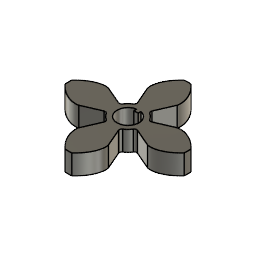
Gear 3 (Autodesk Fusion 360 design; units mm, degrees)
description: Spur Gear; Module: 12.700000; Num Teeth: 4; Pressure Angle: 20.000000; Backlash: 0.00 mm
Autodesk Fusion 360 part; units mm, degrees
sketch "Sketch1" plane through (0, 0, 0) normal (0, 0, 1) x (1, 0, 0) in component "Spur Gear (4 teeth)"
  circle A0 centre (0, 0) radius 10.1092
  circle A1 centre (0, 0) radius 6.35
extrude "Extrude1" add sketch "Sketch1" along normal blind 12.7 in component "Spur Gear (4 teeth)"
sketch "Sketch2" plane through (0, 0, 0) normal (0, 0, 1) x (1, 0, 0) in component "Spur Gear (4 teeth)"
  spline S0 degree 5 poles (21.9128, -9.4616) (21.9552, -9.4799) (22.0407, -9.5141) (22.1712, -9.5583) (22.3491, -9.6037) (22.5768, -9.6426) (22.8081, -9.6692) (23.0414, -9.6889) (23.2758, -9.7048) (23.5109, -9.7174) (23.7467, -9.7262) (23.9837, -9.7295) (24.2219, -9.7262) (24.4615, -9.7158) (24.7023, -9.6987) (24.9439, -9.6758) (25.1862, -9.648) (25.4288, -9.6159) (25.6717, -9.5798) (25.9149, -9.5397) (26.1582, -9.4952) (26.4018, -9.4462) (26.6456, -9.3926) (26.8896, -9.3344) (27.1337, -9.2719) (27.3777, -9.2051) (27.6217, -9.1343) (27.8655, -9.0596) (28.109, -8.9811) (28.3523, -8.8987) (28.5954, -8.8125) (28.838, -8.7225) (29.0803, -8.6286) (29.3222, -8.531) (29.5637, -8.4296) (29.8046, -8.3246) (30.045, -8.216) (30.2848, -8.1038) (30.5239, -7.9882) (30.7623, -7.869) (31.0001, -7.7465) (31.2371, -7.6205) (31.4733, -7.491) (31.7087, -7.3583) (31.9432, -7.2221) (32.1769, -7.0827) (32.4096, -6.9401) (32.6414, -6.7942) (32.8722, -6.6451) (33.1019, -6.4928) (33.3306, -6.3374) (33.5583, -6.1789) (33.7848, -6.0173) (34.0102, -5.8526) (34.2343, -5.6849) (34.4573, -5.5142) (34.6791, -5.3405) (34.8996, -5.1639) (35.1188, -4.9843) (35.3367, -4.8018) (35.5532, -4.6165) (35.7684, -4.4283) (35.9823, -4.2373) (36.1947, -4.0436) (36.4056, -3.847) (36.6151, -3.6477) (36.823, -3.4457) (37.0294, -3.241) (37.2343, -3.0337) (37.4376, -2.8237) (37.6393, -2.6111) (37.7995, -2.4389) (37.9189, -2.3086) (37.9982, -2.2212) (38.0377, -2.1774) knots 0 0 0 0 0 0 0.01428571 0.02857143 0.04285714 0.05714286 0.07142857 0.08571429 0.1 0.11428571 0.12857143 0.14285714 0.15714286 0.17142857 0.18571429 0.2 0.21428571 0.22857143 0.24285714 0.25714286 0.27142857 0.28571429 0.3 0.31428571 0.32857143 0.34285714 0.35714286 0.37142857 0.38571429 0.4 0.41428571 0.42857143 0.44285714 0.45714286 0.47142857 0.48571429 0.5 0.51428571 0.52857143 0.54285714 0.55714286 0.57142857 0.58571429 0.6 0.61428571 0.62857143 0.64285714 0.65714286 0.67142857 0.68571429 0.7 0.71428571 0.72857143 0.74285714 0.75714286 0.77142857 0.78571429 0.8 0.81428571 0.82857143 0.84285714 0.85714286 0.87142857 0.88571429 0.9 0.91428571 0.92857143 0.94285714 0.95714286 0.97142857 0.98571429 1 1 1 1 1 1
  spline S1 degree 5 poles (21.9128, 9.4616) (21.9552, 9.4799) (22.0407, 9.5141) (22.1712, 9.5583) (22.3491, 9.6037) (22.5768, 9.6426) (22.8081, 9.6692) (23.0414, 9.6889) (23.2758, 9.7048) (23.5109, 9.7174) (23.7467, 9.7262) (23.9837, 9.7295) (24.2219, 9.7262) (24.4615, 9.7158) (24.7023, 9.6987) (24.9439, 9.6758) (25.1862, 9.648) (25.4288, 9.6159) (25.6717, 9.5798) (25.9149, 9.5397) (26.1582, 9.4952) (26.4018, 9.4462) (26.6456, 9.3926) (26.8896, 9.3344) (27.1337, 9.2719) (27.3777, 9.2051) (27.6217, 9.1343) (27.8655, 9.0596) (28.109, 8.9811) (28.3523, 8.8987) (28.5954, 8.8125) (28.838, 8.7225) (29.0803, 8.6286) (29.3222, 8.531) (29.5637, 8.4296) (29.8046, 8.3246) (30.045, 8.216) (30.2848, 8.1038) (30.5239, 7.9882) (30.7623, 7.869) (31.0001, 7.7465) (31.2371, 7.6205) (31.4733, 7.491) (31.7087, 7.3583) (31.9432, 7.2221) (32.1769, 7.0827) (32.4096, 6.9401) (32.6414, 6.7942) (32.8722, 6.6451) (33.1019, 6.4928) (33.3306, 6.3374) (33.5583, 6.1789) (33.7848, 6.0173) (34.0102, 5.8526) (34.2343, 5.6849) (34.4573, 5.5142) (34.6791, 5.3405) (34.8996, 5.1639) (35.1188, 4.9843) (35.3367, 4.8018) (35.5532, 4.6165) (35.7684, 4.4283) (35.9823, 4.2373) (36.1947, 4.0436) (36.4056, 3.847) (36.6151, 3.6477) (36.823, 3.4457) (37.0294, 3.241) (37.2343, 3.0337) (37.4376, 2.8237) (37.6393, 2.6111) (37.7995, 2.4389) (37.9189, 2.3086) (37.9982, 2.2212) (38.0377, 2.1774) knots 0 0 0 0 0 0 0.01428571 0.02857143 0.04285714 0.05714286 0.07142857 0.08571429 0.1 0.11428571 0.12857143 0.14285714 0.15714286 0.17142857 0.18571429 0.2 0.21428571 0.22857143 0.24285714 0.25714286 0.27142857 0.28571429 0.3 0.31428571 0.32857143 0.34285714 0.35714286 0.37142857 0.38571429 0.4 0.41428571 0.42857143 0.44285714 0.45714286 0.47142857 0.48571429 0.5 0.51428571 0.52857143 0.54285714 0.55714286 0.57142857 0.58571429 0.6 0.61428571 0.62857143 0.64285714 0.65714286 0.67142857 0.68571429 0.7 0.71428571 0.72857143 0.74285714 0.75714286 0.77142857 0.78571429 0.8 0.81428571 0.82857143 0.84285714 0.85714286 0.87142857 0.88571429 0.9 0.91428571 0.92857143 0.94285714 0.95714286 0.97142857 0.98571429 1 1 1 1 1 1
  arc A0 (38.0377, -2.1774) -> (38.0377, 2.1774) centre (0, 0) ccw
  line L0 (9.2718, -4.0074) -> (21.9128, -9.4616)
  line L1 (9.2718, 4.0074) -> (21.9128, 9.4616)
  line L2 (9.2718, -4.0074) -> (9.2718, 4.0074)
  point P0 (22.9255, -9.6784)
  point P1 (24.0052, -9.7278)
  point P2 (25.1271, -9.6541)
  point P3 (26.2802, -9.4701)
  point P4 (27.4564, -9.1817)
  point P5 (28.6488, -8.792)
  point P6 (29.8509, -8.303)
  point P7 (31.0565, -7.7159)
  point P8 (32.2598, -7.0314)
  point P9 (33.4549, -6.2504)
  point P10 (34.636, -5.3736)
  point P11 (35.7973, -4.4018)
  point P12 (36.9331, -3.336)
  point P13 (22.9255, 9.6784)
  point P14 (24.0052, 9.7278)
  point P15 (25.1271, 9.6541)
  point P16 (26.2802, 9.4701)
  point P17 (27.4564, 9.1817)
  point P18 (28.6488, 8.792)
  point P19 (29.8509, 8.303)
  point P20 (31.0565, 7.7159)
  point P21 (32.2598, 7.0314)
  point P22 (33.4549, 6.2504)
  point P23 (34.636, 5.3736)
  point P24 (35.7973, 4.4018)
  point P25 (36.9331, 3.336)
extrude "Extrude2" add sketch "Sketch2" along normal blind 12.7 in component "Spur Gear (4 teeth)"
fillet "Fillet1" radius 1.5875 2 edges at (9.2795, -4.0107, 6.35) (9.2795, 4.0107, 6.35) in component "Spur Gear (4 teeth)"
pattern_circular "C-Pattern1" count 4 over 360 about axis through (0, 0, 0) along (0, 0, 1) of "Extrude2", "Fillet1" in component "Spur Gear (4 teeth)"
sketch "Sketch3" plane through (0, 0, 0) normal (0, 0, 1) x (1, 0, 0) in component "Spur Gear (4 teeth)"
  circle A0 centre (0, 0) radius 25.4 construction
sketch "Sketch1 (2)" plane through (0, 0, 12.7) normal (0, 0, 1) x (-1, 0, 0)
  arc A0 (-5.2324, 8.6498) -> (-8.6498, 5.2324) centre (0, 0) ccw
  arc A1 (-10.637, 4.5964) -> (-8.6498, 5.2324) centre (-10.0081, 6.054) ccw
  line L0 (-10.637, 4.5964) -> (-21.9128, 9.4616)
  spline S0 degree 5 poles (-21.9128, 9.4616) (-21.9552, 9.4799) (-22.0407, 9.5141) (-22.1712, 9.5583) (-22.3491, 9.6037) (-22.5768, 9.6426) (-22.8081, 9.6692) (-23.0414, 9.6889) (-23.2758, 9.7048) (-23.5109, 9.7174) (-23.7467, 9.7262) (-23.9837, 9.7295) (-24.2219, 9.7262) (-24.4615, 9.7158) (-24.7023, 9.6987) (-24.9439, 9.6758) (-25.1862, 9.648) (-25.4288, 9.6159) (-25.6717, 9.5798) (-25.9149, 9.5397) (-26.1582, 9.4952) (-26.4018, 9.4462) (-26.6456, 9.3926) (-26.8896, 9.3344) (-27.1337, 9.2719) (-27.3777, 9.2051) (-27.6217, 9.1343) (-27.8655, 9.0596) (-28.109, 8.9811) (-28.3523, 8.8987) (-28.5954, 8.8125) (-28.838, 8.7225) (-29.0803, 8.6286) (-29.3222, 8.531) (-29.5637, 8.4296) (-29.8046, 8.3246) (-30.045, 8.216) (-30.2848, 8.1038) (-30.5239, 7.9882) (-30.7623, 7.869) (-31.0001, 7.7465) (-31.2371, 7.6205) (-31.4733, 7.491) (-31.7087, 7.3583) (-31.9432, 7.2221) (-32.1769, 7.0827) (-32.4096, 6.9401) (-32.6414, 6.7942) (-32.8722, 6.6451) (-33.1019, 6.4928) (-33.3306, 6.3374) (-33.5583, 6.1789) (-33.7848, 6.0173) (-34.0102, 5.8526) (-34.2343, 5.6849) (-34.4573, 5.5142) (-34.6791, 5.3405) (-34.8996, 5.1639) (-35.1188, 4.9843) (-35.3367, 4.8018) (-35.5532, 4.6165) (-35.7684, 4.4283) (-35.9823, 4.2373) (-36.1947, 4.0436) (-36.4056, 3.847) (-36.6151, 3.6477) (-36.823, 3.4457) (-37.0294, 3.241) (-37.2343, 3.0337) (-37.4376, 2.8237) (-37.6393, 2.6111) (-37.7995, 2.4389) (-37.9189, 2.3086) (-37.9982, 2.2212) (-38.0377, 2.1774) knots 0 0 0 0 0 0 0.01428571 0.02857143 0.04285714 0.05714286 0.07142857 0.08571429 0.1 0.11428571 0.12857143 0.14285714 0.15714286 0.17142857 0.18571429 0.2 0.21428571 0.22857143 0.24285714 0.25714286 0.27142857 0.28571429 0.3 0.31428571 0.32857143 0.34285714 0.35714286 0.37142857 0.38571429 0.4 0.41428571 0.42857143 0.44285714 0.45714286 0.47142857 0.48571429 0.5 0.51428571 0.52857143 0.54285714 0.55714286 0.57142857 0.58571429 0.6 0.61428571 0.62857143 0.64285714 0.65714286 0.67142857 0.68571429 0.7 0.71428571 0.72857143 0.74285714 0.75714286 0.77142857 0.78571429 0.8 0.81428571 0.82857143 0.84285714 0.85714286 0.87142857 0.88571429 0.9 0.91428571 0.92857143 0.94285714 0.95714286 0.97142857 0.98571429 1 1 1 1 1 1
  arc A2 (-38.0377, 2.1774) -> (-38.0377, -2.1774) centre (0, 0) ccw
  spline S1 degree 5 poles (-38.0377, -2.1774) (-37.9982, -2.2212) (-37.9189, -2.3086) (-37.7995, -2.4389) (-37.6393, -2.6111) (-37.4376, -2.8237) (-37.2343, -3.0337) (-37.0294, -3.241) (-36.823, -3.4457) (-36.6151, -3.6477) (-36.4056, -3.847) (-36.1947, -4.0436) (-35.9823, -4.2373) (-35.7684, -4.4283) (-35.5532, -4.6165) (-35.3367, -4.8018) (-35.1188, -4.9843) (-34.8996, -5.1639) (-34.6791, -5.3405) (-34.4573, -5.5142) (-34.2343, -5.6849) (-34.0102, -5.8526) (-33.7848, -6.0173) (-33.5583, -6.1789) (-33.3306, -6.3374) (-33.1019, -6.4928) (-32.8722, -6.6451) (-32.6414, -6.7942) (-32.4096, -6.9401) (-32.1769, -7.0827) (-31.9432, -7.2221) (-31.7087, -7.3583) (-31.4733, -7.491) (-31.2371, -7.6205) (-31.0001, -7.7465) (-30.7623, -7.869) (-30.5239, -7.9882) (-30.2848, -8.1038) (-30.045, -8.216) (-29.8046, -8.3246) (-29.5637, -8.4296) (-29.3222, -8.531) (-29.0803, -8.6286) (-28.838, -8.7225) (-28.5954, -8.8125) (-28.3523, -8.8987) (-28.109, -8.9811) (-27.8655, -9.0596) (-27.6217, -9.1343) (-27.3777, -9.2051) (-27.1337, -9.2719) (-26.8896, -9.3344) (-26.6456, -9.3926) (-26.4018, -9.4462) (-26.1582, -9.4952) (-25.9149, -9.5397) (-25.6717, -9.5798) (-25.4288, -9.6159) (-25.1862, -9.648) (-24.9439, -9.6758) (-24.7023, -9.6987) (-24.4615, -9.7158) (-24.2219, -9.7262) (-23.9837, -9.7295) (-23.7467, -9.7262) (-23.5109, -9.7174) (-23.2758, -9.7048) (-23.0414, -9.6889) (-22.8081, -9.6692) (-22.5768, -9.6426) (-22.3491, -9.6037) (-22.1712, -9.5583) (-22.0407, -9.5141) (-21.9552, -9.4799) (-21.9128, -9.4616) knots -1 -1 -1 -1 -1 -1 -0.98571429 -0.97142857 -0.95714286 -0.94285714 -0.92857143 -0.91428571 -0.9 -0.88571429 -0.87142857 -0.85714286 -0.84285714 -0.82857143 -0.81428571 -0.8 -0.78571429 -0.77142857 -0.75714286 -0.74285714 -0.72857143 -0.71428571 -0.7 -0.68571429 -0.67142857 -0.65714286 -0.64285714 -0.62857143 -0.61428571 -0.6 -0.58571429 -0.57142857 -0.55714286 -0.54285714 -0.52857143 -0.51428571 -0.5 -0.48571429 -0.47142857 -0.45714286 -0.44285714 -0.42857143 -0.41428571 -0.4 -0.38571429 -0.37142857 -0.35714286 -0.34285714 -0.32857143 -0.31428571 -0.3 -0.28571429 -0.27142857 -0.25714286 -0.24285714 -0.22857143 -0.21428571 -0.2 -0.18571429 -0.17142857 -0.15714286 -0.14285714 -0.12857143 -0.11428571 -0.1 -0.08571429 -0.07142857 -0.05714286 -0.04285714 -0.02857143 -0.01428571 0 0 0 0 0 0
  line L1 (-21.9128, -9.4616) -> (-10.637, -4.5964)
  arc A3 (-8.6498, -5.2324) -> (-10.637, -4.5964) centre (-10.0081, -6.054) ccw
  arc A4 (-8.6498, -5.2324) -> (-5.2324, -8.6498) centre (0, 0) ccw
  arc A5 (-4.5964, -10.637) -> (-5.2324, -8.6498) centre (-6.054, -10.0081) ccw
  line L2 (-4.5964, -10.637) -> (-9.4616, -21.9128)
  spline S2 degree 5 poles (-9.4616, -21.9128) (-9.4799, -21.9552) (-9.5141, -22.0407) (-9.5583, -22.1712) (-9.6037, -22.3491) (-9.6426, -22.5768) (-9.6692, -22.8081) (-9.6889, -23.0414) (-9.7048, -23.2758) (-9.7174, -23.5109) (-9.7262, -23.7467) (-9.7295, -23.9837) (-9.7262, -24.2219) (-9.7158, -24.4615) (-9.6987, -24.7023) (-9.6758, -24.9439) (-9.648, -25.1862) (-9.6159, -25.4288) (-9.5798, -25.6717) (-9.5397, -25.9149) (-9.4952, -26.1582) (-9.4462, -26.4018) (-9.3926, -26.6456) (-9.3344, -26.8896) (-9.2719, -27.1337) (-9.2051, -27.3777) (-9.1343, -27.6217) (-9.0596, -27.8655) (-8.9811, -28.109) (-8.8987, -28.3523) (-8.8125, -28.5954) (-8.7225, -28.838) (-8.6286, -29.0803) (-8.531, -29.3222) (-8.4296, -29.5637) (-8.3246, -29.8046) (-8.216, -30.045) (-8.1038, -30.2848) (-7.9882, -30.5239) (-7.869, -30.7623) (-7.7465, -31.0001) (-7.6205, -31.2371) (-7.491, -31.4733) (-7.3583, -31.7087) (-7.2221, -31.9432) (-7.0827, -32.1769) (-6.9401, -32.4096) (-6.7942, -32.6414) (-6.6451, -32.8722) (-6.4928, -33.1019) (-6.3374, -33.3306) (-6.1789, -33.5583) (-6.0173, -33.7848) (-5.8526, -34.0102) (-5.6849, -34.2343) (-5.5142, -34.4573) (-5.3405, -34.6791) (-5.1639, -34.8996) (-4.9843, -35.1188) (-4.8018, -35.3367) (-4.6165, -35.5532) (-4.4283, -35.7684) (-4.2373, -35.9823) (-4.0436, -36.1947) (-3.847, -36.4056) (-3.6477, -36.6151) (-3.4457, -36.823) (-3.241, -37.0294) (-3.0337, -37.2343) (-2.8237, -37.4376) (-2.6111, -37.6393) (-2.4389, -37.7995) (-2.3086, -37.9189) (-2.2212, -37.9982) (-2.1774, -38.0377) knots 0 0 0 0 0 0 0.01428571 0.02857143 0.04285714 0.05714286 0.07142857 0.08571429 0.1 0.11428571 0.12857143 0.14285714 0.15714286 0.17142857 0.18571429 0.2 0.21428571 0.22857143 0.24285714 0.25714286 0.27142857 0.28571429 0.3 0.31428571 0.32857143 0.34285714 0.35714286 0.37142857 0.38571429 0.4 0.41428571 0.42857143 0.44285714 0.45714286 0.47142857 0.48571429 0.5 0.51428571 0.52857143 0.54285714 0.55714286 0.57142857 0.58571429 0.6 0.61428571 0.62857143 0.64285714 0.65714286 0.67142857 0.68571429 0.7 0.71428571 0.72857143 0.74285714 0.75714286 0.77142857 0.78571429 0.8 0.81428571 0.82857143 0.84285714 0.85714286 0.87142857 0.88571429 0.9 0.91428571 0.92857143 0.94285714 0.95714286 0.97142857 0.98571429 1 1 1 1 1 1
  arc A6 (-2.1774, -38.0377) -> (2.1774, -38.0377) centre (0, 0) ccw
  spline S3 degree 5 poles (2.1774, -38.0377) (2.2212, -37.9982) (2.3086, -37.9189) (2.4389, -37.7995) (2.6111, -37.6393) (2.8237, -37.4376) (3.0337, -37.2343) (3.241, -37.0294) (3.4457, -36.823) (3.6477, -36.6151) (3.847, -36.4056) (4.0436, -36.1947) (4.2373, -35.9823) (4.4283, -35.7684) (4.6165, -35.5532) (4.8018, -35.3367) (4.9843, -35.1188) (5.1639, -34.8996) (5.3405, -34.6791) (5.5142, -34.4573) (5.6849, -34.2343) (5.8526, -34.0102) (6.0173, -33.7848) (6.1789, -33.5583) (6.3374, -33.3306) (6.4928, -33.1019) (6.6451, -32.8722) (6.7942, -32.6414) (6.9401, -32.4096) (7.0827, -32.1769) (7.2221, -31.9432) (7.3583, -31.7087) (7.491, -31.4733) (7.6205, -31.2371) (7.7465, -31.0001) (7.869, -30.7623) (7.9882, -30.5239) (8.1038, -30.2848) (8.216, -30.045) (8.3246, -29.8046) (8.4296, -29.5637) (8.531, -29.3222) (8.6286, -29.0803) (8.7225, -28.838) (8.8125, -28.5954) (8.8987, -28.3523) (8.9811, -28.109) (9.0596, -27.8655) (9.1343, -27.6217) (9.2051, -27.3777) (9.2719, -27.1337) (9.3344, -26.8896) (9.3926, -26.6456) (9.4462, -26.4018) (9.4952, -26.1582) (9.5397, -25.9149) (9.5798, -25.6717) (9.6159, -25.4288) (9.648, -25.1862) (9.6758, -24.9439) (9.6987, -24.7023) (9.7158, -24.4615) (9.7262, -24.2219) (9.7295, -23.9837) (9.7262, -23.7467) (9.7174, -23.5109) (9.7048, -23.2758) (9.6889, -23.0414) (9.6692, -22.8081) (9.6426, -22.5768) (9.6037, -22.3491) (9.5583, -22.1712) (9.5141, -22.0407) (9.4799, -21.9552) (9.4616, -21.9128) knots -1 -1 -1 -1 -1 -1 -0.98571429 -0.97142857 -0.95714286 -0.94285714 -0.92857143 -0.91428571 -0.9 -0.88571429 -0.87142857 -0.85714286 -0.84285714 -0.82857143 -0.81428571 -0.8 -0.78571429 -0.77142857 -0.75714286 -0.74285714 -0.72857143 -0.71428571 -0.7 -0.68571429 -0.67142857 -0.65714286 -0.64285714 -0.62857143 -0.61428571 -0.6 -0.58571429 -0.57142857 -0.55714286 -0.54285714 -0.52857143 -0.51428571 -0.5 -0.48571429 -0.47142857 -0.45714286 -0.44285714 -0.42857143 -0.41428571 -0.4 -0.38571429 -0.37142857 -0.35714286 -0.34285714 -0.32857143 -0.31428571 -0.3 -0.28571429 -0.27142857 -0.25714286 -0.24285714 -0.22857143 -0.21428571 -0.2 -0.18571429 -0.17142857 -0.15714286 -0.14285714 -0.12857143 -0.11428571 -0.1 -0.08571429 -0.07142857 -0.05714286 -0.04285714 -0.02857143 -0.01428571 0 0 0 0 0 0
  line L3 (9.4616, -21.9128) -> (4.5964, -10.637)
  arc A7 (5.2324, -8.6498) -> (4.5964, -10.637) centre (6.054, -10.0081) ccw
  arc A8 (5.2324, -8.6498) -> (8.6498, -5.2324) centre (0, 0) ccw
  arc A9 (10.637, -4.5964) -> (8.6498, -5.2324) centre (10.0081, -6.054) ccw
  line L4 (10.637, -4.5964) -> (21.9128, -9.4616)
  spline S4 degree 5 poles (21.9128, -9.4616) (21.9552, -9.4799) (22.0407, -9.5141) (22.1712, -9.5583) (22.3491, -9.6037) (22.5768, -9.6426) (22.8081, -9.6692) (23.0414, -9.6889) (23.2758, -9.7048) (23.5109, -9.7174) (23.7467, -9.7262) (23.9837, -9.7295) (24.2219, -9.7262) (24.4615, -9.7158) (24.7023, -9.6987) (24.9439, -9.6758) (25.1862, -9.648) (25.4288, -9.6159) (25.6717, -9.5798) (25.9149, -9.5397) (26.1582, -9.4952) (26.4018, -9.4462) (26.6456, -9.3926) (26.8896, -9.3344) (27.1337, -9.2719) (27.3777, -9.2051) (27.6217, -9.1343) (27.8655, -9.0596) (28.109, -8.9811) (28.3523, -8.8987) (28.5954, -8.8125) (28.838, -8.7225) (29.0803, -8.6286) (29.3222, -8.531) (29.5637, -8.4296) (29.8046, -8.3246) (30.045, -8.216) (30.2848, -8.1038) (30.5239, -7.9882) (30.7623, -7.869) (31.0001, -7.7465) (31.2371, -7.6205) (31.4733, -7.491) (31.7087, -7.3583) (31.9432, -7.2221) (32.1769, -7.0827) (32.4096, -6.9401) (32.6414, -6.7942) (32.8722, -6.6451) (33.1019, -6.4928) (33.3306, -6.3374) (33.5583, -6.1789) (33.7848, -6.0173) (34.0102, -5.8526) (34.2343, -5.6849) (34.4573, -5.5142) (34.6791, -5.3405) (34.8996, -5.1639) (35.1188, -4.9843) (35.3367, -4.8018) (35.5532, -4.6165) (35.7684, -4.4283) (35.9823, -4.2373) (36.1947, -4.0436) (36.4056, -3.847) (36.6151, -3.6477) (36.823, -3.4457) (37.0294, -3.241) (37.2343, -3.0337) (37.4376, -2.8237) (37.6393, -2.6111) (37.7995, -2.4389) (37.9189, -2.3086) (37.9982, -2.2212) (38.0377, -2.1774) knots 0 0 0 0 0 0 0.01428571 0.02857143 0.04285714 0.05714286 0.07142857 0.08571429 0.1 0.11428571 0.12857143 0.14285714 0.15714286 0.17142857 0.18571429 0.2 0.21428571 0.22857143 0.24285714 0.25714286 0.27142857 0.28571429 0.3 0.31428571 0.32857143 0.34285714 0.35714286 0.37142857 0.38571429 0.4 0.41428571 0.42857143 0.44285714 0.45714286 0.47142857 0.48571429 0.5 0.51428571 0.52857143 0.54285714 0.55714286 0.57142857 0.58571429 0.6 0.61428571 0.62857143 0.64285714 0.65714286 0.67142857 0.68571429 0.7 0.71428571 0.72857143 0.74285714 0.75714286 0.77142857 0.78571429 0.8 0.81428571 0.82857143 0.84285714 0.85714286 0.87142857 0.88571429 0.9 0.91428571 0.92857143 0.94285714 0.95714286 0.97142857 0.98571429 1 1 1 1 1 1
  arc A10 (38.0377, -2.1774) -> (38.0377, 2.1774) centre (0, 0) ccw
  spline S5 degree 5 poles (38.0377, 2.1774) (37.9982, 2.2212) (37.9189, 2.3086) (37.7995, 2.4389) (37.6393, 2.6111) (37.4376, 2.8237) (37.2343, 3.0337) (37.0294, 3.241) (36.823, 3.4457) (36.6151, 3.6477) (36.4056, 3.847) (36.1947, 4.0436) (35.9823, 4.2373) (35.7684, 4.4283) (35.5532, 4.6165) (35.3367, 4.8018) (35.1188, 4.9843) (34.8996, 5.1639) (34.6791, 5.3405) (34.4573, 5.5142) (34.2343, 5.6849) (34.0102, 5.8526) (33.7848, 6.0173) (33.5583, 6.1789) (33.3306, 6.3374) (33.1019, 6.4928) (32.8722, 6.6451) (32.6414, 6.7942) (32.4096, 6.9401) (32.1769, 7.0827) (31.9432, 7.2221) (31.7087, 7.3583) (31.4733, 7.491) (31.2371, 7.6205) (31.0001, 7.7465) (30.7623, 7.869) (30.5239, 7.9882) (30.2848, 8.1038) (30.045, 8.216) (29.8046, 8.3246) (29.5637, 8.4296) (29.3222, 8.531) (29.0803, 8.6286) (28.838, 8.7225) (28.5954, 8.8125) (28.3523, 8.8987) (28.109, 8.9811) (27.8655, 9.0596) (27.6217, 9.1343) (27.3777, 9.2051) (27.1337, 9.2719) (26.8896, 9.3344) (26.6456, 9.3926) (26.4018, 9.4462) (26.1582, 9.4952) (25.9149, 9.5397) (25.6717, 9.5798) (25.4288, 9.6159) (25.1862, 9.648) (24.9439, 9.6758) (24.7023, 9.6987) (24.4615, 9.7158) (24.2219, 9.7262) (23.9837, 9.7295) (23.7467, 9.7262) (23.5109, 9.7174) (23.2758, 9.7048) (23.0414, 9.6889) (22.8081, 9.6692) (22.5768, 9.6426) (22.3491, 9.6037) (22.1712, 9.5583) (22.0407, 9.5141) (21.9552, 9.4799) (21.9128, 9.4616) knots -1 -1 -1 -1 -1 -1 -0.98571429 -0.97142857 -0.95714286 -0.94285714 -0.92857143 -0.91428571 -0.9 -0.88571429 -0.87142857 -0.85714286 -0.84285714 -0.82857143 -0.81428571 -0.8 -0.78571429 -0.77142857 -0.75714286 -0.74285714 -0.72857143 -0.71428571 -0.7 -0.68571429 -0.67142857 -0.65714286 -0.64285714 -0.62857143 -0.61428571 -0.6 -0.58571429 -0.57142857 -0.55714286 -0.54285714 -0.52857143 -0.51428571 -0.5 -0.48571429 -0.47142857 -0.45714286 -0.44285714 -0.42857143 -0.41428571 -0.4 -0.38571429 -0.37142857 -0.35714286 -0.34285714 -0.32857143 -0.31428571 -0.3 -0.28571429 -0.27142857 -0.25714286 -0.24285714 -0.22857143 -0.21428571 -0.2 -0.18571429 -0.17142857 -0.15714286 -0.14285714 -0.12857143 -0.11428571 -0.1 -0.08571429 -0.07142857 -0.05714286 -0.04285714 -0.02857143 -0.01428571 0 0 0 0 0 0
  line L5 (21.9128, 9.4616) -> (10.637, 4.5964)
  arc A11 (8.6498, 5.2324) -> (10.637, 4.5964) centre (10.0081, 6.054) ccw
  arc A12 (8.6498, 5.2324) -> (5.2324, 8.6498) centre (0, 0) ccw
  arc A13 (4.5964, 10.637) -> (5.2324, 8.6498) centre (6.054, 10.0081) ccw
  line L6 (4.5964, 10.637) -> (9.4616, 21.9128)
  spline S6 degree 5 poles (9.4616, 21.9128) (9.4799, 21.9552) (9.5141, 22.0407) (9.5583, 22.1712) (9.6037, 22.3491) (9.6426, 22.5768) (9.6692, 22.8081) (9.6889, 23.0414) (9.7048, 23.2758) (9.7174, 23.5109) (9.7262, 23.7467) (9.7295, 23.9837) (9.7262, 24.2219) (9.7158, 24.4615) (9.6987, 24.7023) (9.6758, 24.9439) (9.648, 25.1862) (9.6159, 25.4288) (9.5798, 25.6717) (9.5397, 25.9149) (9.4952, 26.1582) (9.4462, 26.4018) (9.3926, 26.6456) (9.3344, 26.8896) (9.2719, 27.1337) (9.2051, 27.3777) (9.1343, 27.6217) (9.0596, 27.8655) (8.9811, 28.109) (8.8987, 28.3523) (8.8125, 28.5954) (8.7225, 28.838) (8.6286, 29.0803) (8.531, 29.3222) (8.4296, 29.5637) (8.3246, 29.8046) (8.216, 30.045) (8.1038, 30.2848) (7.9882, 30.5239) (7.869, 30.7623) (7.7465, 31.0001) (7.6205, 31.2371) (7.491, 31.4733) (7.3583, 31.7087) (7.2221, 31.9432) (7.0827, 32.1769) (6.9401, 32.4096) (6.7942, 32.6414) (6.6451, 32.8722) (6.4928, 33.1019) (6.3374, 33.3306) (6.1789, 33.5583) (6.0173, 33.7848) (5.8526, 34.0102) (5.6849, 34.2343) (5.5142, 34.4573) (5.3405, 34.6791) (5.1639, 34.8996) (4.9843, 35.1188) (4.8018, 35.3367) (4.6165, 35.5532) (4.4283, 35.7684) (4.2373, 35.9823) (4.0436, 36.1947) (3.847, 36.4056) (3.6477, 36.6151) (3.4457, 36.823) (3.241, 37.0294) (3.0337, 37.2343) (2.8237, 37.4376) (2.6111, 37.6393) (2.4389, 37.7995) (2.3086, 37.9189) (2.2212, 37.9982) (2.1774, 38.0377) knots 0 0 0 0 0 0 0.01428571 0.02857143 0.04285714 0.05714286 0.07142857 0.08571429 0.1 0.11428571 0.12857143 0.14285714 0.15714286 0.17142857 0.18571429 0.2 0.21428571 0.22857143 0.24285714 0.25714286 0.27142857 0.28571429 0.3 0.31428571 0.32857143 0.34285714 0.35714286 0.37142857 0.38571429 0.4 0.41428571 0.42857143 0.44285714 0.45714286 0.47142857 0.48571429 0.5 0.51428571 0.52857143 0.54285714 0.55714286 0.57142857 0.58571429 0.6 0.61428571 0.62857143 0.64285714 0.65714286 0.67142857 0.68571429 0.7 0.71428571 0.72857143 0.74285714 0.75714286 0.77142857 0.78571429 0.8 0.81428571 0.82857143 0.84285714 0.85714286 0.87142857 0.88571429 0.9 0.91428571 0.92857143 0.94285714 0.95714286 0.97142857 0.98571429 1 1 1 1 1 1
  arc A14 (2.1774, 38.0377) -> (-2.1774, 38.0377) centre (0, 0) ccw
  spline S7 degree 5 poles (-2.1774, 38.0377) (-2.2212, 37.9982) (-2.3086, 37.9189) (-2.4389, 37.7995) (-2.6111, 37.6393) (-2.8237, 37.4376) (-3.0337, 37.2343) (-3.241, 37.0294) (-3.4457, 36.823) (-3.6477, 36.6151) (-3.847, 36.4056) (-4.0436, 36.1947) (-4.2373, 35.9823) (-4.4283, 35.7684) (-4.6165, 35.5532) (-4.8018, 35.3367) (-4.9843, 35.1188) (-5.1639, 34.8996) (-5.3405, 34.6791) (-5.5142, 34.4573) (-5.6849, 34.2343) (-5.8526, 34.0102) (-6.0173, 33.7848) (-6.1789, 33.5583) (-6.3374, 33.3306) (-6.4928, 33.1019) (-6.6451, 32.8722) (-6.7942, 32.6414) (-6.9401, 32.4096) (-7.0827, 32.1769) (-7.2221, 31.9432) (-7.3583, 31.7087) (-7.491, 31.4733) (-7.6205, 31.2371) (-7.7465, 31.0001) (-7.869, 30.7623) (-7.9882, 30.5239) (-8.1038, 30.2848) (-8.216, 30.045) (-8.3246, 29.8046) (-8.4296, 29.5637) (-8.531, 29.3222) (-8.6286, 29.0803) (-8.7225, 28.838) (-8.8125, 28.5954) (-8.8987, 28.3523) (-8.9811, 28.109) (-9.0596, 27.8655) (-9.1343, 27.6217) (-9.2051, 27.3777) (-9.2719, 27.1337) (-9.3344, 26.8896) (-9.3926, 26.6456) (-9.4462, 26.4018) (-9.4952, 26.1582) (-9.5397, 25.9149) (-9.5798, 25.6717) (-9.6159, 25.4288) (-9.648, 25.1862) (-9.6758, 24.9439) (-9.6987, 24.7023) (-9.7158, 24.4615) (-9.7262, 24.2219) (-9.7295, 23.9837) (-9.7262, 23.7467) (-9.7174, 23.5109) (-9.7048, 23.2758) (-9.6889, 23.0414) (-9.6692, 22.8081) (-9.6426, 22.5768) (-9.6037, 22.3491) (-9.5583, 22.1712) (-9.5141, 22.0407) (-9.4799, 21.9552) (-9.4616, 21.9128) knots -1 -1 -1 -1 -1 -1 -0.98571429 -0.97142857 -0.95714286 -0.94285714 -0.92857143 -0.91428571 -0.9 -0.88571429 -0.87142857 -0.85714286 -0.84285714 -0.82857143 -0.81428571 -0.8 -0.78571429 -0.77142857 -0.75714286 -0.74285714 -0.72857143 -0.71428571 -0.7 -0.68571429 -0.67142857 -0.65714286 -0.64285714 -0.62857143 -0.61428571 -0.6 -0.58571429 -0.57142857 -0.55714286 -0.54285714 -0.52857143 -0.51428571 -0.5 -0.48571429 -0.47142857 -0.45714286 -0.44285714 -0.42857143 -0.41428571 -0.4 -0.38571429 -0.37142857 -0.35714286 -0.34285714 -0.32857143 -0.31428571 -0.3 -0.28571429 -0.27142857 -0.25714286 -0.24285714 -0.22857143 -0.21428571 -0.2 -0.18571429 -0.17142857 -0.15714286 -0.14285714 -0.12857143 -0.11428571 -0.1 -0.08571429 -0.07142857 -0.05714286 -0.04285714 -0.02857143 -0.01428571 0 0 0 0 0 0
  line L7 (-9.4616, 21.9128) -> (-4.5964, 10.637)
  arc A15 (-5.2324, 8.6498) -> (-4.5964, 10.637) centre (-6.054, 10.0081) ccw
  circle A16 centre (0, 0) radius 6.35
  circle A17 centre (0, 0) radius 7
  circle A18 centre (0, 0) radius 6.35
  line L8 (1.4, -6.8586) -> (1.4, -5.1)
  line L9 (1.4, -5.1) -> (-1.4, -5.1)
  line L10 (-1.4, -5.1) -> (-1.4, -6.8586)
  line L11 (0, -9) -> (0, 8.2774)
  point P0 (0, -7)
  dimension "d17" = 14
  dimension "d18" = 2.8
  dimension "d19" = 1.9
  constraint coincident A0.centre A2.centre
  constraint coincident A17 L8.start
  constraint vertical L8
  constraint perpendicular L8 L9
  constraint coincident A17 L10.end
  constraint perpendicular L9 L10
  constraint perpendicular L9 L11
  constraint symmetric L8 L10 L11
  constraint coincident A17 P0
  constraint coincident L11 P0
  constraint coincident A0.centre L11
  measures "d17" diameter of A17
  measures "d18" distance of L8 L10
  measures "d19" distance of L9 P0
extrude "Extrude3" cut sketch "Sketch1 (2)" against normal blind 12.7 contours A16 A17 A18 L8 L11 | A16 A17 A18 L10 L11 | A16 A17 A18 L8 L11 | A16 A17 A18 L10 L11 in component "Spur Gear (4 teeth)"
extrude "Extrude4" add sketch "Sketch1 (2)" against normal up to surface (12.7 mm away) contours A16 A17 A18 L8 L11 | A16 A18 L8 L9 L11 | A16 A18 L9 L10 L11 | A16 A17 A18 L10 L11 picked at (1.2459, -6.4442) picked at (0.7792, -5.4935) picked at (-0.7792, -5.4935) picked at (-1.2459, -6.4442) in component "Spur Gear (4 teeth)"
component "Spur Gear (4 teeth)" placed x (1, 0, 0) y (0, 1, 0) z (0, 0, 1) at (0, 0, 0)
